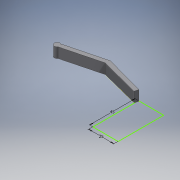
# Autodesk Inventor part: arm1
Saved by Autodesk Inventor 2020 (Build 240168000, 168)
## iProperties
Created: 2020-02-04
Part Number: arm1
Material: Generic
Document SubType Name: Modeling
Designer: Wes
Density: 1 g/cm^3
Appearance: Default
Author: Wes
Autodesk Inventor part; units mm, degrees
ref_plane "YZ Plane" through (0, 0, 0) normal (1, 0, 0) x (0, 1, 0)
ref_plane "XZ Plane" through (0, 0, 0) normal (0, 1, 0) x (-1, 0, 0)
ref_plane "XY Plane" through (0, 0, 0) normal (0, 0, 1) x (1, 0, 0)
sketch "Sketch1 - gripper" plane through (0, 0, 0) normal (0, 0, 1) x (1, 0, 0)
  line L0 (0, 0) -> (-10, -38.7298)
  line L1 (-10, -38.7298) -> (0, -38.7298) construction
  line L2 (-10, -38.7298) -> (0, -77.4597)
  line L3 (0, 0) -> (-3.873, 1)
  line L4 (-3.873, 1) -> (-14.3579, -37.8519)
  line L5 (-14.3579, -37.8519) -> (-3.873, -78.4597)
  line L6 (-3.873, -78.4597) -> (0, -77.4597)
  circle A0 centre (-1.9365, -77.9597) radius 2.75
  point P0 (-4.3448, -76.6321)
  point P1 (-0.4719, -75.6321)
  dimension "d18" = 40
  dimension "d19" = 40
  dimension "d20" = 4
  dimension "d21" = 5.5
  constraints: 14 end point, 2 perpendicular, 1 centre point, 1 horizontal, 1 midpoint
  measures "d18" distance of L0.start L0.end
  measures "d19" distance of L0.end L2.end
  measures "d20" distance of L0.start L3.end
  measures "d21" diameter of A0
extrude "Extrusion1" add sketch "Sketch1 - gripper" along normal blind 10
sketch "Sketch3" plane through (0, 0, 0) normal (0, 0, -1) x (-1, 0, 0)
  line L0 (10, -38.7298) -> (0, 0) construction
  line L1 (3.873, 1) -> (14.3579, -37.8519) projected
  line L2 (4.1429, 0) -> (-40.8571, 0)
  line L3 (-40.8571, 0) -> (-40.8571, 25)
  line L4 (-40.8571, 25) -> (4.1429, 25)
  line L5 (4.1429, 25) -> (4.1429, 0)
  dimension "d22" = 45
  dimension "d23" = 25
  constraints: 8 end point, 2 perpendicular, 1 horizontal, 1 point on line
  measures "d22" distance of L2.start L2.end
  measures "d23" distance of L2.end L3.end
body "Solid2"
